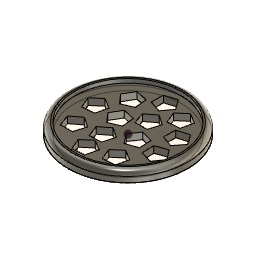
7.6 appearance (Autodesk Fusion 360 design; units mm, degrees)
Autodesk Fusion 360 part; units mm, degrees
sketch "Sketch1" plane through (0, 0, 0) normal (0, 0, 1) x (1, 0, 0)
  circle A0 centre (0, 0) radius 45
  circle A1 centre (0, 0) radius 40
  dimension "d1" = 90
  dimension "d2" = -5
  constraint coincident A0.centre A1.centre
  measures "d1" diameter of A0
extrude "Extrude1" add sketch "Sketch1" along normal blind 8
extrude "Extrude2" add sketch "Sketch1" along normal blind 5 contours A1
sketch "Sketch2" plane through (0, 0, 5) normal (0, 0, 1) x (-1, 0, 0)
  line L0 (9.7065, -15.2032) -> (10.5595, -24.1789)
  line L1 (10.5595, -24.1789) -> (19.3595, -26.1413)
  line L2 (19.3595, -26.1413) -> (23.9453, -18.3784)
  line L3 (23.9453, -18.3784) -> (17.9794, -11.6183)
  line L4 (17.9794, -11.6183) -> (9.7065, -15.2032)
  line L5 (2.3064, 1.7998) -> (3.1593, -7.176)
  line L6 (16.5451, -1.3755) -> (10.5792, 5.3847)
  line L7 (10.5792, 5.3847) -> (2.3064, 1.7998)
  line L8 (3.1593, -7.176) -> (11.9594, -9.1384)
  line L9 (11.9594, -9.1384) -> (16.5451, -1.3755)
  line L10 (-0.1005, -5.1751) -> (-9.1149, -5.3544)
  line L11 (-11.73, -13.983) -> (-4.3318, -19.1365)
  line L12 (-4.3318, -19.1365) -> (2.8556, -13.6929)
  line L13 (-9.1149, -5.3544) -> (-11.73, -13.983)
  line L14 (2.8556, -13.6929) -> (-0.1005, -5.1751)
  line L15 (17.5268, 24.1869) -> (14.993, 15.534)
  line L16 (22.4394, 10.4504) -> (29.5752, 15.9614)
  line L17 (29.5752, 15.9614) -> (26.5391, 24.451)
  line L18 (14.993, 15.534) -> (22.4394, 10.4504)
  line L19 (26.5391, 24.451) -> (17.5268, 24.1869)
  line L20 (33.7221, -3.6823) -> (30.2498, 4.6384)
  line L21 (30.2498, 4.6384) -> (21.2633, 3.9073)
  line L22 (19.1816, -4.8653) -> (26.8816, -9.5559)
  line L23 (21.2633, 3.9073) -> (19.1816, -4.8653)
  line L24 (26.8816, -9.5559) -> (33.7221, -3.6823)
  line L25 (7.0524, -33.7264) -> (7.1423, -24.7107)
  line L26 (7.1423, -24.7107) -> (-1.4044, -21.8392)
  line L27 (-1.5498, -36.427) -> (7.0524, -33.7264)
  line L28 (-1.4044, -21.8392) -> (-6.7764, -29.0802)
  line L29 (-6.7764, -29.0802) -> (-1.5498, -36.427)
  line L30 (8.7825, 20.5049) -> (-0.2283, 20.1944)
  line L31 (4.7548, 6.4834) -> (11.8623, 12.031)
  line L32 (11.8623, 12.031) -> (8.7825, 20.5049)
  line L33 (-0.2283, 20.1944) -> (-2.7176, 11.5287)
  line L34 (-2.7176, 11.5287) -> (4.7548, 6.4834)
  line L35 (-9.6613, 12.6209) -> (-18.1524, 9.5888)
  line L36 (-4.1538, 5.4824) -> (-9.6613, 12.6209)
  line L37 (-17.8926, 0.5764) -> (-9.241, -1.9616)
  line L38 (-9.241, -1.9616) -> (-4.1538, 5.4824)
  line L39 (-18.1524, 9.5888) -> (-17.8926, 0.5764)
  line L40 (-29.0638, -18.1025) -> (-20.4014, -15.6016)
  line L41 (-20.1031, -6.5904) -> (-28.5811, -3.522)
  line L42 (-28.5811, -3.522) -> (-34.1191, -10.6369)
  line L43 (-34.1191, -10.6369) -> (-29.0638, -18.1025)
  line L44 (-20.4014, -15.6016) -> (-20.1031, -6.5904)
  line L45 (-20.2979, 29.9068) -> (-22.3795, 21.1342)
  line L46 (-14.6796, 16.4435) -> (-7.8391, 22.3171)
  line L47 (-22.3795, 21.1342) -> (-14.6796, 16.4435)
  line L48 (-7.8391, 22.3171) -> (-11.3114, 30.6379)
  line L49 (-11.3114, 30.6379) -> (-20.2979, 29.9068)
  line L50 (-22.4664, 11.7936) -> (-31.0997, 14.393)
  line L51 (-31.0997, 14.393) -> (-36.2397, 6.9854)
  line L52 (-30.783, -0.1921) -> (-22.2706, 2.7796)
  line L53 (-22.2706, 2.7796) -> (-22.4664, 11.7936)
  line L54 (-36.2397, 6.9854) -> (-30.783, -0.1921)
  line L55 (-4.3507, 26.0684) -> (3.3493, 21.3777)
  line L56 (10.1898, 27.2513) -> (6.7174, 35.5721)
  line L57 (3.3493, 21.3777) -> (10.1898, 27.2513)
  line L58 (-2.2691, 34.841) -> (-4.3507, 26.0684)
  line L59 (6.7174, 35.5721) -> (-2.2691, 34.841)
  line L60 (-15.175, -31.8449) -> (-8.3345, -25.9713)
  line L61 (-11.8069, -17.6506) -> (-20.7934, -18.3817)
  line L62 (-22.875, -27.1543) -> (-15.175, -31.8449)
  line L63 (-8.3345, -25.9713) -> (-11.8069, -17.6506)
  line L64 (-20.7934, -18.3817) -> (-22.875, -27.1543)
  point P0 (16.31, -19.104)
  point P1 (8.9099, -2.1011)
  point P2 (-4.4843, -11.4684)
  point P3 (22.2147, 18.1167)
  point P4 (26.2597, -1.9116)
  point P5 (0.8928, -29.1567)
  point P6 (4.4907, 14.1485)
  point P7 (-11.8202, 5.2614)
  point P8 (-26.4537, -10.8907)
  point P9 (-15.3015, 24.0879)
  point P10 (-28.5719, 7.1519)
  point P11 (6.7127, 26.555)
  point P12 (2.7273, 29.0221)
  point P13 (-15.797, -24.2006)
extrude "Extrude3" cut sketch "Sketch2" against normal through all
fillet "Fillet1" radius 3.793 1 edges at (-41.9547, -16.2727, 8)
